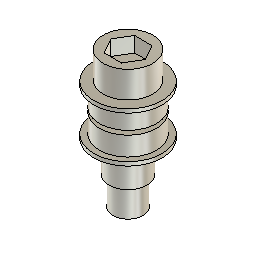
Mark III Core XY assembly v25 (Autodesk Fusion 360 archive; units mm, degrees)
design "8mm pulley low"
Autodesk Fusion 360 part; units mm, degrees
(part 1 of 2)
sketch "Sketch1" plane through (0, 0, 0) normal (0, 0, 1) x (1, 0, 0)
sketch "Sketch2" plane through (0, 0, 0) normal (0, 0, 1) x (1, 0, 0)
  circle A0 centre (0, 0) radius 4
  dimension "d4" = 8
  constraint coincident A0.centre origin
  measures "d4" diameter of A0
extrude "Extrude2" add sketch "Sketch2" along normal blind 27 contours A0 picked at (1.42018, -0.528552) makes body 1
sketch "Sketch3" plane through (0, 0, 27) normal (0, 0, 1) x (-1, 0, 0)
  circle A0 centre (0, 0) radius 4
  circle A1 centre (0, 0) radius 6.5
  dimension "d7" = 13
  constraint concentric A0 A1
  measures "d7" diameter of A1
extrude "Extrude3" add sketch "Sketch3" along normal blind 10 contours A0 | A1 picked at (-0.705317, 0.780795) picked at (5.627575, -0.521648) bodies 1
sketch "Sketch4" plane through (0, 0, 37) normal (0, 0, 1) x (-1, 0, 0)
  circle A0 centre (0, 0) radius 6.5
  line L0 (-4.618187, 0.0754) -> (-2.374392, -3.961767)
  line L1 (-2.374392, -3.961767) -> (2.243795, -4.037167)
  line L2 (2.243795, -4.037167) -> (4.618187, -0.0754)
  line L3 (4.618187, -0.0754) -> (2.374392, 3.961767)
  line L4 (2.374392, 3.961767) -> (-2.243795, 4.037167)
  line L5 (-2.243795, 4.037167) -> (-4.618187, 0.0754)
  dimension "d10" = 4
  constraint coincident A0.centre origin
  measures "d10" distance of A0.centre L5
extrude "Extrude4" cut sketch "Sketch4" against normal blind 7 contours L0 L1 L2 L3 L4 L5 picked at (-1.539396, 0.025133) bodies 1
thread "Thread1" [suppressed]
sketch "Sketch5" plane through (0, 0, 37) normal (0, 0, 1) x (-1, 0, 0)
  circle A0 centre (-1.50985, 25.955849) radius 4
  circle A1 centre (-1.50985, 25.955849) radius 8
  circle A2 centre (-1.50985, 25.955849) radius 9
  dimension "d13" = 8
  dimension "d14" = 16
  dimension "d15" = 18
  constraint concentric A0 A1
  constraint concentric A1 A2
  measures "d13" diameter of A0
  measures "d14" diameter of A1
  measures "d15" diameter of A2
sketch "Sketch6" plane through (0, 0, 42) normal (0, 0, 1) x (-1, 0, 0)
  circle A0 centre (-1.50985, 25.955849) radius 4
  circle A1 centre (-1.50985, 25.955849) radius 8
  circle A2 centre (-1.50985, 25.955849) radius 5
  circle A3 centre (-1.50985, 25.955849) radius 7.5
  dimension "d20" = 10
  dimension "d21" = 15
  constraint concentric A0 A2
  constraint concentric A2 A3
  measures "d20" diameter of A2
  measures "d21" diameter of A3
extrude "Extrude7" add sketch "Sketch6" against normal blind 5 separate body contours A3 picked at (5.110278, 25.33484) makes body 2
extrude "Extrude8" add sketch "Sketch5" against normal blind 1 separate body contours A2 picked at (7.093525, 25.111277) makes body 3
sketch "Sketch7" plane through (0, 0, 42) normal (0, 0, 1) x (1, 0, 0)
extrude "Extrude9" add sketch "Sketch5" against normal blind 1 contours A1 picked at (5.11214, 25.35968) bodies 2 3
move_face "OffsetFaces1" offset 5 1 faces at (-3.138201, -25.707446, 37) on bodies 2
copy_body "CopyPasteBodies1" bodies 2 makes body 4
move_body "Move1" bodies 4 to x (-1, 0, 0) y (0, 1, 0) z (0, 0, -1) at (3.0197, 0, 84.5)
move_body "Move2" bodies 1 to x (1, 0, 0) y (0, 1, 0) z (0, 0, 1) at (44, -25, 0)
move_body "Align1" bodies 1 to x (1, 0, 0) y (0, 1, 0) z (0, 0, 1) at (-42.49015, -0.955849, 45.732394)
move_body "Move3" bodies 2 4 to x (1, 0, 0) y (0, 1, 0) z (0, 0, 1) at (0, 0, 24)
move_body "Move4" bodies 2 to x (1, 0, 0) y (0, 1, 0) z (0, 0, 1) at (0, 0, -55)
sketch "Sketch8" plane through (0, 0, 45.732394) normal (0, 0, -1) x (1, 0, 0)
  circle A0 centre (1.50914, 25.951936) radius 4
  circle A1 centre (1.50914, 25.951936) radius 5
  circle A2 centre (1.50985, 25.955849) radius 4
  dimension "d29" = 8
  dimension "d30" = 10
  constraint concentric A0 A1
  measures "d29" diameter of A0
  measures "d30" diameter of A1
extrude "Extrude10" add sketch "Sketch6" along normal blind 1 separate body contours A2 picked at (3.138201, 25.707446) makes body 5
move_body "Move5" bodies 5 to x (1, 0, 0) y (0, 1, 0) z (0, 0, 1) at (0, 0, 23.5)
move_body "Move6" bodies 2 to x (1, 0, 0) y (0, 1, 0) z (0, 0, 1) at (0, 0, 54.4)
sketch "Sketch9" plane through (0, 0, 45.732394) normal (0, 0, -1) x (1, 0, 0)
  circle A0 centre (1.50974, 25.955286) radius 4
  circle A1 centre (1.50974, 25.955286) radius 5
  circle A2 centre (1.50985, 25.955849) radius 4
  dimension "d34" = 8
  dimension "d35" = 10
  constraint concentric A0 A1
  measures "d34" diameter of A0
  measures "d35" diameter of A1
extrude "Extrude11" add sketch "Sketch8" against normal blind 10 separate body contours A1 picked at (-0.514215, 21.757072) makes body 6
move_body "Move7" bodies 6 to x (1, 0, 0) y (0, 1, 0) z (0, 0, 1) at (0, 0, 3.5)
move_face "OffsetFaces3" offset -3 1 faces at (-0.514215, -21.757072, 49.232394) on bodies 6
extrude "Extrude12" cut 1 faces at (1.715297, -21.12893, 82.732394) along direction (0, 0, -1) blind 3 on bodies 1 bodies 1
move_face "OffsetFaces4" offset 2 1 faces at (2.883587, -26.892448, 45.732394) on bodies 1
extrude "Extrude13" add 1 faces at (-0.514215, -21.757072, 52.232394) along direction (0, 0, -1) blind 1.0883 on bodies 6 bodies 6 2 4 5 1
ref_plane "WorkPlane1" through (0, -2, 0) normal (0, 1, 0) x (0, 0, 1)
sketch "Sketch10" plane through (0, -2, 0) normal (0, 1, 0) x (1, 0, 0)
  line L0 (6.509162, -59.23223) -> (6.509162, -51.144083)
  constraint vertical L0
sketch "Sketch11" plane through (0, 0, 0) normal (0, 1, 0) x (1, 0, 0)
combine "Combine1" [suppressed]
named bodies: "pulley low"

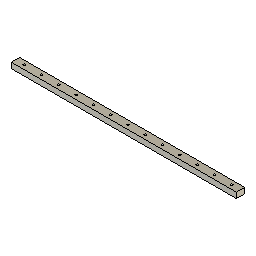
design "rail"
Autodesk Fusion 360 part; units mm, degrees
sketch "Sketch1" plane through (0, 0, 0) normal (0, 0, 1) x (1, 0, 0)
  line L0 (0, 0) -> (325, 0)
  line L1 (325, 0) -> (325, -12)
  line L2 (325, -12) -> (0, -12)
  line L3 (0, -12) -> (0, 0)
  circle A0 centre (12.5, -6) radius 1.5
  circle A1 centre (37.5, -6) radius 1.5
  circle A2 centre (62.5, -6) radius 1.5
  circle A3 centre (87.5, -6) radius 1.5
  circle A4 centre (137.5, -6) radius 1.5
  circle A5 centre (112.5, -6) radius 1.5
  circle A6 centre (262.5, -6) radius 1.5
  circle A7 centre (162.5, -6) radius 1.5
  circle A8 centre (212.5, -6) radius 1.5
  circle A9 centre (237.5, -6) radius 1.5
  circle A10 centre (287.5, -6) radius 1.5
  circle A11 centre (187.5, -6) radius 1.5
  circle A12 centre (312.5, -6) radius 1.5
  point P0 (287.5, -6)
  point P1 (262.5, -6)
  point P2 (187.5, -6)
  point P3 (112.5, -6)
  point P4 (37.5, -6)
  point P5 (62.5, -6)
  point P6 (87.5, -6)
  point P7 (162.5, -6)
  point P8 (137.5, -6)
  point P9 (212.5, -6)
  point P10 (237.5, -6)
  point P11 (12.5, -6)
  point P12 (112.5, -6)
  point P13 (87.5, -6)
  point P14 (137.5, -6)
  point P15 (287.5, -6)
  point P16 (262.5, -6)
  point P17 (187.5, -6)
  point P18 (237.5, -6)
  point P19 (262.5, -6)
  point P20 (287.5, -6)
  point P21 (237.5, -6)
  point P22 (162.5, -6)
  point P23 (212.5, -6)
  point P24 (312.5, -6)
  point P25 (312.5, -6)
  point P26 (312.5, -6)
  dimension "d1" = 325
  dimension "d2" = 12
  dimension "d6" = 25
  dimension "d12" = 25
  dimension "d13" = 25
  dimension "d14" = 25
  dimension "d15" = 25
  dimension "d16" = 25
  dimension "d17" = 25
  dimension "d18" = 25
  dimension "d19" = 3
  dimension "d20" = 3
  dimension "d21" = 3
  dimension "d22" = 25
  dimension "d23" = 25
  dimension "d24" = 3
  dimension "d25" = 3
  dimension "d26" = 3
  dimension "d27" = 25
  dimension "d28" = 25
  dimension "d29" = 25
  dimension "d30" = 25
  dimension "d31" = 3
  dimension "d32" = 3
  dimension "d33" = 3
  dimension "d34" = 25
  dimension "d35" = 25
  dimension "d36" = 3
  dimension "d37" = 3
  dimension "d38" = 3
  dimension "d39" = 3
  constraint horizontal L0
  constraint vertical L1
  constraint horizontal L2
  constraint vertical L3
  constraint coincident L0.start L3.end
  constraint coincident P11 A0.centre
  constraint coincident P4 A1.centre
  constraint coincident P5 A2.centre
  constraint coincident P13 P6
  constraint coincident P12 P3
  constraint coincident P14 P8
  constraint coincident P22 P7
  constraint coincident P17 P2
  constraint coincident P23 P9
  constraint coincident P21 P18
  constraint coincident P19 P16
  constraint coincident P20 P15
  constraint coincident P26 P25
  measures "d1" distance of L0.start L0.end
  measures "d2" distance of L0.start L2.end
  measures "d6" distance of P20 P19
  measures "d12" distance of P4 P5
  measures "d13" distance of P5 P13
  measures "d14" distance of P12 P14
  measures "d15" distance of P22 P14
  measures "d16" distance of P17 P23
  measures "d17" distance of P23 P21
  measures "d18" distance of P4 P11
  measures "d19" diameter of A0
  measures "d20" diameter of A1
  measures "d21" diameter of A2
  measures "d22" distance of P12 P14
  measures "d23" distance of P12 P13
  measures "d24" diameter of A3
  measures "d25" diameter of A5
  measures "d26" diameter of A4
  measures "d27" distance of P17 P23
  measures "d28" distance of P21 P23
  measures "d29" distance of P20 P19
  measures "d30" distance of P17 P22
  measures "d31" diameter of A7
  measures "d32" diameter of A11
  measures "d33" diameter of A8
  measures "d34" distance of P19 P20
  measures "d35" distance of P21 P19
  measures "d36" diameter of A9
  measures "d37" diameter of A6
  measures "d38" diameter of A10
  measures "d39" diameter of A12
extrude "Extrude1" add sketch "Sketch1" along normal blind 8

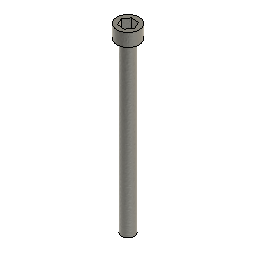
design "long stepper allen bolt"
Autodesk Fusion 360 part; units mm, degrees
sketch "Sketch1" plane through (0, 0, 0) normal (0, 0, 1) x (1, 0, 0)
  circle A0 centre (0, 0) radius 2.5
  dimension "d1" = 5
  constraint coincident A0.centre origin
  measures "d1" diameter of A0
extrude "Extrude1" add sketch "Sketch1" along normal blind 65
sketch "Sketch2" plane through (0, 0, 65) normal (0, 0, 1) x (-1, 0, 0)
  circle A0 centre (0, 0) radius 2.5
  circle A1 centre (0, 0) radius 4.3
  dimension "d4" = 8.6
  constraint coincident A0.centre A1.centre
  measures "d4" diameter of A1
extrude "Extrude2" add sketch "Sketch2" along normal blind 5 contours A0 | A1
sketch "Sketch3" plane through (0, 0, 70) normal (0, 0, 1) x (-1, 0, 0)
  circle A0 centre (0, 0) radius 4.3
  line L0 (-2.8697, 0.3419) -> (-1.7309, -2.3143)
  line L1 (-1.7309, -2.3143) -> (1.1388, -2.6561)
  line L2 (1.1388, -2.6561) -> (2.8697, -0.3419)
  line L3 (2.8697, -0.3419) -> (1.7309, 2.3143)
  line L4 (1.7309, 2.3143) -> (-1.1388, 2.6561)
  line L5 (-1.1388, 2.6561) -> (-2.8697, 0.3419)
  dimension "d7" = 2.5028
  constraint coincident A0.centre origin
  measures "d7" distance of A0.centre L5
extrude "Extrude3" cut sketch "Sketch3" against normal blind 4 contours L0 L1 L2 L3 L4 L5

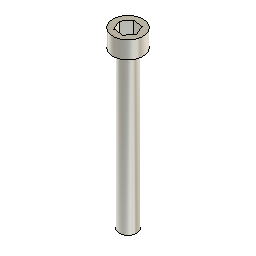
design "45mm short  stepper allen bolt"
Autodesk Fusion 360 part; units mm, degrees
sketch "Sketch1" plane through (0, 0, 0) normal (0, 0, 1) x (1, 0, 0)
  circle A0 centre (0, 0) radius 2.5
  dimension "d1" = 5
  constraint coincident A0.centre origin
  measures "d1" diameter of A0
sketch "Sketch2" plane through (0, 0, 65) normal (0, 0, 1) x (-1, 0, 0)
  circle A0 centre (0, 0) radius 2.5
  circle A1 centre (0, 0) radius 4.3
  dimension "d4" = 8.6
  constraint coincident A0.centre A1.centre
  measures "d4" diameter of A1
extrude "Extrude4" add sketch "Sketch1" along normal blind 45 makes body 1
extrude "Extrude2" add sketch "Sketch2" along normal blind 5 contours A0 | A1 makes body 2
sketch "Sketch3" plane through (0, 0, 70) normal (0, 0, 1) x (-1, 0, 0)
  circle A0 centre (0, 0) radius 4.3
  line L0 (-2.8697, 0.3419) -> (-1.7309, -2.3143)
  line L1 (-1.7309, -2.3143) -> (1.1388, -2.6561)
  line L2 (1.1388, -2.6561) -> (2.8697, -0.3419)
  line L3 (2.8697, -0.3419) -> (1.7309, 2.3143)
  line L4 (1.7309, 2.3143) -> (-1.1388, 2.6561)
  line L5 (-1.1388, 2.6561) -> (-2.8697, 0.3419)
  dimension "d7" = 2.5028
  constraint coincident A0.centre origin
  measures "d7" distance of A0.centre L5
extrude "Extrude3" cut sketch "Sketch3" against normal blind 4 contours L0 L1 L2 L3 L4 L5 bodies 2
move_body "Align1" bodies 2 to x (1, 0, 0) y (0, 1, 0) z (0, 0, 1) at (0, 0, -20)

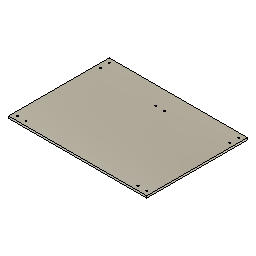
design "bottom plate"
Autodesk Fusion 360 part; units mm, degrees
sketch "Sketch1" plane through (0, 0, 0) normal (0, 0, 1) x (1, 0, 0)
  line L0 (14.0053, -24.8588) -> (645.8303, -24.8588)
  line L1 (645.8303, -24.8588) -> (645.8303, -485.2338)
  line L2 (645.8303, -485.2338) -> (14.0053, -485.2338)
  line L3 (14.0053, -485.2338) -> (14.0053, -24.8588)
  dimension "d1" = 631.825
  dimension "d2" = 460.375
  constraint horizontal L0
  constraint vertical L1
  constraint horizontal L2
  constraint vertical L3
  measures "d1" distance of L0.start L0.end
  measures "d2" distance of L0.start L2.end
extrude "Extrude1" add sketch "Sketch1" along normal blind 9.525
sketch "Sketch2" plane through (0, 0, 19.05) normal (0, 0, 1) x (-1, 0, 0)
  circle A0 centre (-559.9411, 33.0388) radius 2
  circle A1 centre (-607.0811, 33.0388) radius 2
  circle A2 centre (-610.8303, 63.0463) radius 3.5
  circle A3 centre (-48.9178, 458.0463) radius 3.5
  circle A4 centre (-610.9178, 458.0463) radius 3.5
  circle A5 centre (-349.9178, 108.3588) radius 3.5
  circle A6 centre (-309.9178, 108.3588) radius 3.5
  circle A7 centre (-625.8303, 84.8588) radius 3.5
  circle A8 centre (-625.8303, 44.8588) radius 3.5
  circle A9 centre (-34.0053, 84.8588) radius 3.5
  circle A10 centre (-34.0053, 44.8588) radius 3.5
  circle A11 centre (-594.8678, 98.3622) radius 3.5
  circle A12 centre (-48.9178, 63.0463) radius 3.5
  circle A13 centre (-76.3246, 82.1788) radius 3.5
  circle A14 centre (-583.5111, 82.1788) radius 3.5
  circle A15 centre (-64.9678, 98.3204) radius 3.5
  circle A16 centre (-625.8303, 465.2338) radius 3.5
  circle A17 centre (-585.8303, 465.2338) radius 3.5
  circle A18 centre (-74.0053, 465.2338) radius 3.5
  circle A19 centre (-34.0053, 465.2338) radius 3.5
  circle A20 centre (-559.9411, 80.1788) radius 2
  circle A21 centre (-607.0811, 80.1788) radius 2
  circle A22 centre (-583.5111, 56.6088) radius 3.5
  circle A23 centre (-99.8946, 80.1788) radius 2
  circle A24 centre (-99.8946, 33.0388) radius 2
  circle A25 centre (-76.3246, 56.6088) radius 3.5
  circle A26 centre (-52.7546, 33.0388) radius 2
  line L0 (-14.0053, 24.8588) -> (-14.0053, 485.2338)
  line L1 (-14.0053, 485.2338) -> (-94.0053, 485.2338)
  line L2 (-94.0053, 485.2338) -> (-94.0053, 445.2338)
  line L3 (-94.0053, 445.2338) -> (-92.5053, 445.2338)
  arc A27 (-77.5053, 430.2338) -> (-92.5053, 445.2338) centre (-92.5053, 430.2338) ccw
  line L4 (-77.5053, 430.2338) -> (-77.5053, 108.3588)
  arc A28 (-97.5053, 88.3588) -> (-77.5053, 108.3588) centre (-97.5053, 108.3588) ccw
  line L5 (-97.5053, 88.3588) -> (-269.9178, 88.3588)
  arc A29 (-289.9178, 108.3588) -> (-269.9178, 88.3588) centre (-269.9178, 108.3588) ccw
  line L6 (-289.9178, 108.3588) -> (-289.9178, 128.3588)
  line L7 (-289.9178, 128.3588) -> (-369.9178, 128.3588)
  line L8 (-369.9178, 128.3588) -> (-369.9178, 108.3588)
  arc A30 (-389.9178, 88.3588) -> (-369.9178, 108.3588) centre (-389.9178, 108.3588) ccw
  line L9 (-389.9178, 88.3588) -> (-562.3303, 88.3588)
  arc A31 (-582.3303, 108.3588) -> (-562.3303, 88.3588) centre (-562.3303, 108.3588) ccw
  line L10 (-582.3303, 108.3588) -> (-582.3303, 430.2338)
  arc A32 (-567.3303, 445.2338) -> (-582.3303, 430.2338) centre (-567.3303, 430.2338) ccw
  line L11 (-567.3303, 445.2338) -> (-565.8303, 445.2338)
  line L12 (-565.8303, 445.2338) -> (-565.8303, 485.2338)
  line L13 (-565.8303, 485.2338) -> (-645.8303, 485.2338)
  line L14 (-645.8303, 485.2338) -> (-645.8303, 24.8588)
  line L15 (-645.8303, 24.8588) -> (-14.0053, 24.8588)
  point P0 (-34.0053, 44.8588)
  point P1 (-34.0053, 84.8588)
  point P2 (-349.9178, 108.3588)
  point P3 (-309.9178, 108.3588)
  point P4 (-625.8303, 84.8588)
  point P5 (-625.8303, 44.8588)
  point P6 (-625.8303, 465.2338)
  point P7 (-585.8303, 465.2338)
  point P8 (-34.0053, 465.2338)
  point P9 (-74.0053, 465.2338)
  constraint coincident P0 A10.centre
  constraint coincident P1 A9.centre
  constraint coincident P2 A5.centre
  constraint coincident P3 A6.centre
  constraint coincident P4 A7.centre
  constraint coincident P5 A8.centre
  constraint coincident P6 A16.centre
  constraint coincident P7 A17.centre
  constraint coincident P8 A19.centre
  constraint coincident P9 A18.centre
hole "Hole1" at (34.0053, -465.2338, 19.05) direction (0, 0, -1) diameter 7 depth 60 tip angle 118
hole "Hole2" at (74.0053, -465.2338, 19.05) at (34.0053, -44.8588, 19.05) at (34.0053, -84.8588, 19.05) at (625.8303, -44.8588, 19.05) at (625.8303, -84.8588, 19.05) direction (0, 0, -1) diameter 7 depth 60 tip angle 118
hole "Hole3" at (625.8303, -465.2338, 19.05) at (585.8303, -465.2338, 19.05) direction (0, 0, -1) diameter 7 depth 60 tip angle 118
hole "Hole4" at (309.9178, -108.3588, 19.05) at (349.9178, -108.3588, 19.05) direction (0, 0, -1) diameter 7 depth 60 tip angle 118

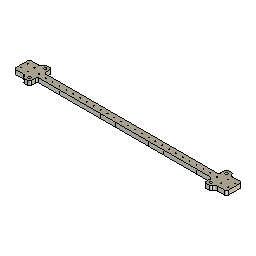
design "Mark III core xy  bridge"
Autodesk Fusion 360 part; units mm, degrees
sketch "Sketch2" plane through (0, 0, 0) normal (0, 0, 1) x (1, 0, 0)
sketch "Sketch5" plane through (0, 0, 9.525) normal (0, 0, 1) x (-1, 0, 0)
sketch "Sketch30" plane through (0, 0, 9.525) normal (0, 0, 1) x (-1, 0, 0)
  line L0 (-255, 10) -> (255, 10)
  line L1 (255, -10) -> (-255, -10)
  line L2 (275, 22.5) -> (310, 22.5)
  line L3 (310, 22.5) -> (310, -22.5)
  line L4 (310, -22.5) -> (275, -22.5)
  line L5 (-310, 22.5) -> (-275, 22.5)
  line L6 (-275, -22.5) -> (-310, -22.5)
  line L7 (-310, -22.5) -> (-310, 22.5)
  line L8 (-275, 22.5) -> (-275, 27.5)
  line L9 (-270, 32.5) -> (-260, 32.5)
  line L10 (-255, 27.5) -> (-255, 10)
  line L11 (-275, -22.5) -> (-275, -27.5)
  line L12 (-270, -32.5) -> (-260, -32.5)
  line L13 (-255, -27.5) -> (-255, -10)
  line L14 (275, -22.5) -> (275, -27.5)
  line L15 (270, -32.5) -> (260, -32.5)
  line L16 (255, -27.5) -> (255, -10)
  line L17 (275, 22.5) -> (275, 27.5)
  line L18 (270, 32.5) -> (260, 32.5)
  line L19 (255, 27.5) -> (255, 10)
  arc A0 (-260, -32.5) -> (-255, -27.5) centre (-260, -27.5) ccw
  arc A1 (-255, 27.5) -> (-260, 32.5) centre (-260, 27.5) ccw
  arc A2 (255, -27.5) -> (260, -32.5) centre (260, -27.5) ccw
  arc A3 (260, 32.5) -> (255, 27.5) centre (260, 27.5) ccw
  arc A4 (275, 27.5) -> (270, 32.5) centre (270, 27.5) ccw
  arc A5 (270, -32.5) -> (275, -27.5) centre (270, -27.5) ccw
  arc A6 (-275, -27.5) -> (-270, -32.5) centre (-270, -27.5) ccw
  arc A7 (-270, 32.5) -> (-275, 27.5) centre (-270, 27.5) ccw
  point P0 (292.5, 0)
  point P1 (-292.5, 0)
  point P2 (-20, 0)
  point P3 (-40, 0)
  point P4 (-100, 0)
  point P5 (-60, 0)
  point P6 (-80, 0)
  point P7 (-60, 0)
  point P8 (-160, 0)
  point P9 (-120, 0)
  point P10 (-220, 0)
  point P11 (-180, 0)
  point P12 (-140, 0)
  point P13 (-200, 0)
  point P14 (-120, 0)
  point P15 (-180, 0)
  point P16 (-240, 0)
  point P17 (-220, 0)
  point P18 (-220, 0)
  point P19 (220, 0)
  point P20 (260, 0)
  point P21 (120, 0)
  point P22 (40, 0)
  point P23 (160, 0)
  point P24 (200, 0)
  point P25 (240, 0)
  point P26 (180, 0)
  point P27 (260, 0)
  point P28 (20, 0)
  point P29 (40, 0)
  point P30 (200, 0)
  point P31 (60, 0)
  point P32 (140, 0)
  point P33 (80, 0)
  point P34 (40, 0)
  point P35 (100, 0)
  point P36 (140, 0)
  point P37 (80, 0)
  point P38 (240, 0)
  point P39 (220, 0)
  point P40 (180, 0)
  point P41 (160, 0)
  point P42 (120, 0)
  point P43 (100, 0)
  point P44 (60, 0)
  point P45 (20, 0)
  point P46 (-80, 0)
  point P47 (-100, 0)
  point P48 (-140, 0)
  point P49 (-160, 0)
  point P50 (-200, 0)
  point P51 (-240, 0)
  point P52 (-260, 0)
  point P53 (-260, 0)
  point P54 (292.5, 0)
  point P55 (282.5, -10)
  point P56 (302.5, -10)
  point P57 (302.5, 10)
  point P58 (282.5, 10)
  point P59 (-302.5, -10)
  point P60 (-282.5, -10)
  point P61 (-282.5, 10)
  point P62 (-302.5, 10)
  point P63 (-275, 32.5)
  point P64 (-255, 32.5)
  point P65 (-275, -32.5)
  point P66 (-255, -32.5)
  point P67 (275, -32.5)
  point P68 (255, -32.5)
  point P69 (275, 32.5)
  point P70 (255, 32.5)
  dimension "d349" = 35
  dimension "d350" = 45
  dimension "d351" = 35
  dimension "d352" = 45
  dimension "d353" = 20
  dimension "d354" = 20
  dimension "d355" = 20
  dimension "d356" = 20
  dimension "d357" = 20
  dimension "d358" = 20
  dimension "d359" = 20
  dimension "d360" = 20
  dimension "d361" = 20
  dimension "d363" = 20
  dimension "d364" = 20
  dimension "d365" = 20
  dimension "d366" = 20
  dimension "d367" = 20
  dimension "d368" = 20
  dimension "d369" = 20
  dimension "d370" = 20
  dimension "d371" = 20
  dimension "d372" = 20
  dimension "d373" = 20
  dimension "d374" = 20
  dimension "d375" = 20
  dimension "d376" = 10
  dimension "d377" = 20
  dimension "d378" = 10
  dimension "d379" = 20
  dimension "d380" = 10
  dimension "d381" = 20
  dimension "d382" = 10
  dimension "d383" = 20
  dimension "d384" = 5
  dimension "d385" = 5
  constraint parallel L0 L1
  constraint horizontal L0
  constraint perpendicular L2 L3
  constraint parallel L2 L4
  constraint horizontal L2
  constraint parallel L5 L6
  constraint horizontal L5
  constraint coincident P7 P5
  constraint coincident P14 P9
  constraint coincident P15 P11
  constraint coincident P18 P17
  constraint coincident P27 P20
  constraint coincident P30 P24
  constraint coincident P36 P32
  constraint coincident P37 P33
  constraint coincident P34 P29
  constraint coincident P38 P25
  constraint coincident P39 P19
  constraint coincident P40 P26
  constraint coincident P41 P23
  constraint coincident P42 P21
  constraint coincident P43 P35
  constraint coincident P44 P31
  constraint coincident P45 P28
  constraint coincident P46 P6
  constraint coincident P47 P4
  constraint coincident P48 P12
  constraint coincident P49 P8
  constraint coincident P50 P13
  constraint coincident P51 P16
  constraint coincident P53 P52
  constraint coincident P54 P0
  constraint perpendicular L5 L8
  constraint perpendicular L8 L9
  constraint perpendicular L0 L10
  constraint perpendicular L6 L11
  constraint perpendicular L11 L12
  constraint perpendicular L1 L13
  constraint perpendicular L4 L14
  constraint perpendicular L14 L15
  constraint perpendicular L1 L16
  constraint perpendicular L1 L17
  constraint perpendicular L17 L18
  constraint perpendicular L0 L19
  constraint coincident P66 L12
  constraint coincident P66 L13
  constraint tangent L12 A0
  constraint tangent L13 A0
  constraint coincident P64 L9
  constraint coincident P64 L10
  constraint tangent L9 A1
  constraint tangent L10 A1
  constraint coincident P68 L15
  constraint coincident P68 L16
  constraint tangent L15 A2
  constraint tangent L16 A2
  constraint equal A1 A2
  constraint coincident P70 L18
  constraint coincident P70 L19
  constraint tangent L18 A3
  constraint tangent L19 A3
  constraint equal A1 A3
  constraint coincident P69 L17
  constraint coincident P69 L18
  constraint tangent L17 A4
  constraint tangent L18 A4
  constraint equal A1 A4
  constraint coincident P67 L14
  constraint coincident P67 L15
  constraint tangent L14 A5
  constraint tangent L15 A5
  constraint equal A1 A5
  constraint coincident P65 L11
  constraint coincident P65 L12
  constraint tangent L11 A6
  constraint tangent L12 A6
  constraint equal A1 A6
  constraint coincident P63 L8
  constraint coincident P63 L9
  constraint tangent L8 A7
  constraint tangent L9 A7
  constraint equal A1 A7
  measures "d349" distance of L3.end L4.end
  measures "d350" distance of L2.end L3.end
  measures "d351" distance of L6.start L6.end
  measures "d352" distance of L5.end L6.start
  measures "d353" distance of origin P2
  measures "d354" distance of P2 P3
  measures "d355" distance of P7 P46
  measures "d356" distance of P47 P46
  measures "d357" distance of P14 P48
  measures "d358" distance of P49 P48
  measures "d359" distance of P15 P50
  measures "d360" distance of P18 P50
  measures "d361" distance of P51 P18
  measures "d363" distance of P27 P38
  measures "d364" distance of P39 P38
  measures "d365" distance of P30 P40
  measures "d366" distance of P41 P40
  measures "d367" distance of P42 P36
  measures "d368" distance of P42 P43
  measures "d369" distance of P44 P37
  measures "d370" distance of P31 P34
  measures "d371" distance of P34 P45
  measures "d372" distance of P55 P56
  measures "d373" distance of P56 P57
  measures "d374" distance of P59 P60
  measures "d375" distance of P60 P61
  measures "d376" distance of L5.end P63
  measures "d377" distance of P63 P64
  measures "d378" distance of L6.start P65
  measures "d379" distance of P65 P66
  measures "d380" distance of L4.end P67
  measures "d381" distance of P67 P68
  measures "d382" distance of L2.start P69
  measures "d383" distance of P69 P70
  measures "d384" radius of A0
  measures "d385" radius of A1
extrude "Extrude17" add sketch "Sketch30" along normal blind 12.7 makes body 1
hole "Hole31" at (-265, -23, 0) direction (0, 0, 1) diameter 7 depth 200 tip angle 118 bodies 1
hole "Hole32" at (-264.95, 22.9974, 0) direction (0, 0, 1) diameter 7 depth 200 tip angle 118 bodies 1
hole "Hole33" at (265, -22.9937, 0) at (265, 23, 0) direction (0, 0, 1) diameter 7 depth 200 tip angle 118 bodies 1
hole "Hole34" at (-302.5, -10, 9.525) direction (0, 0, 1) diameter 3 depth 200 tip angle 118 bodies 1
hole "Hole35" at (-302.5, 10, 9.525) at (-282.5, 10, 9.525) at (-282.5, -10, 9.525) at (302.5, -10, 9.525) at (282.5, -10, 9.525) at (282.5, 10, 9.525) at (302.5, 10, 9.525) direction (0, 0, 1) diameter 3 depth 200 tip angle 118 bodies 1
hole "Hole36" at (260, 0, 9.525) direction (0, 0, 1) diameter 2.5 depth 200 tip angle 118 bodies 1
hole "Hole37" at (240, 0, 9.525) at (220, 0, 9.525) at (200, 0, 9.525) at (180, 0, 9.525) at (160, 0, 9.525) at (140, 0, 9.525) at (120, 0, 9.525) at (100, 0, 9.525) at (80, 0, 9.525) at (60, 0, 9.525) at (40, 0, 9.525) at (20, 0, 9.525) at (-20, 0, 9.525) at (-40, 0, 9.525) at (-60, 0, 9.525) at (-80, 0, 9.525) at (-100, 0, 9.525) at (-260, 0, 9.525) at (-240, 0, 9.525) at (-220, 0, 9.525) at (-200, 0, 9.525) at (-180, 0, 9.525) at (-160, 0, 9.525) at (-140, 0, 9.525) at (-120, 0, 9.525) direction (0, 0, 1) diameter 2.5 depth 200 tip angle 118 bodies 1
hole "Hole38" at (0, 0, 9.525) direction (0, 0, 1) diameter 2.5 depth 200 tip angle 118 bodies 1
thread "Thread1" [suppressed]
fillet "Fillet1" radius 5 4 edges at (-310, 22.5, 15.875) (310, 22.5, 15.875) (310, -22.5, 15.875) (-310, -22.5, 15.875) on bodies 1
fillet "Fillet2" radius 5 4 edges at (-255, -10, 15.875) (255, -10, 15.875) (-255, 10, 15.875) (255, 10, 15.875) on bodies 1
move_body "Move32" bodies 1 to x (1, 0, 0) y (0, 1, 0) z (0, 0, 1) at (0, 0, 20)
sketch "Sketch31" plane through (0, 0, 29.525) normal (0, 0, -1) x (1, 0, 0)
  arc A0 (-305, 22.5) -> (-310, 17.5) centre (-305, 17.5) ccw
  line L0 (-310, 17.5) -> (-310, -17.5)
  arc A1 (-310, -17.5) -> (-305, -22.5) centre (-305, -17.5) ccw
  line L1 (-305, -22.5) -> (-275, -22.5)
  line L2 (-275, -22.5) -> (-275, -27.5)
  arc A2 (-275, -27.5) -> (-270, -32.5) centre (-270, -27.5) ccw
  line L3 (-270, -32.5) -> (-260, -32.5)
  arc A3 (-260, -32.5) -> (-255, -27.5) centre (-260, -27.5) ccw
  line L4 (-255, -27.5) -> (-255, -15)
  arc A4 (-250, -10) -> (-255, -15) centre (-250, -15) ccw
  line L5 (-250, -10) -> (250, -10)
  arc A5 (255, -15) -> (250, -10) centre (250, -15) ccw
  line L6 (255, -15) -> (255, -27.5)
  arc A6 (255, -27.5) -> (260, -32.5) centre (260, -27.5) ccw
  line L7 (260, -32.5) -> (270, -32.5)
  arc A7 (270, -32.5) -> (275, -27.5) centre (270, -27.5) ccw
  line L8 (275, -27.5) -> (275, -22.5)
  line L9 (275, -22.5) -> (305, -22.5)
  arc A8 (305, -22.5) -> (310, -17.5) centre (305, -17.5) ccw
  line L10 (310, -17.5) -> (310, 17.5)
  arc A9 (310, 17.5) -> (305, 22.5) centre (305, 17.5) ccw
  line L11 (305, 22.5) -> (275, 22.5)
  line L12 (275, 22.5) -> (275, 27.5)
  arc A10 (275, 27.5) -> (270, 32.5) centre (270, 27.5) ccw
  line L13 (270, 32.5) -> (260, 32.5)
  arc A11 (260, 32.5) -> (255, 27.5) centre (260, 27.5) ccw
  line L14 (255, 27.5) -> (255, 15)
  arc A12 (250, 10) -> (255, 15) centre (250, 15) ccw
  line L15 (250, 10) -> (-250, 10)
  arc A13 (-255, 15) -> (-250, 10) centre (-250, 15) ccw
  line L16 (-255, 15) -> (-255, 27.5)
  arc A14 (-255, 27.5) -> (-260, 32.5) centre (-260, 27.5) ccw
  line L17 (-260, 32.5) -> (-270, 32.5)
  arc A15 (-270, 32.5) -> (-275, 27.5) centre (-270, 27.5) ccw
  line L18 (-275, 27.5) -> (-275, 22.5)
  line L19 (-275, 22.5) -> (-305, 22.5)
  circle A16 centre (0, 0) radius 1.25
  circle A17 centre (-140, 0) radius 1.25
  circle A18 centre (-180, 0) radius 1.25
  circle A19 centre (-220, 0) radius 1.25
  circle A20 centre (-260, 0) radius 1.25
  circle A21 centre (-80, 0) radius 1.25
  circle A22 centre (-40, 0) radius 1.25
  circle A23 centre (20, 0) radius 1.25
  circle A24 centre (60, 0) radius 1.25
  circle A25 centre (100, 0) radius 1.25
  circle A26 centre (140, 0) radius 1.25
  circle A27 centre (180, 0) radius 1.25
  circle A28 centre (220, 0) radius 1.25
  circle A29 centre (240, 0) radius 1.25
  circle A30 centre (200, 0) radius 1.25
  circle A31 centre (160, 0) radius 1.25
  circle A32 centre (120, 0) radius 1.25
  circle A33 centre (80, 0) radius 1.25
  circle A34 centre (40, 0) radius 1.25
  circle A35 centre (-20, 0) radius 1.25
  circle A36 centre (-60, 0) radius 1.25
  circle A37 centre (-100, 0) radius 1.25
  circle A38 centre (-240, 0) radius 1.25
  circle A39 centre (-200, 0) radius 1.25
  circle A40 centre (-160, 0) radius 1.25
  circle A41 centre (-120, 0) radius 1.25
  circle A42 centre (260, 0) radius 1.25
  circle A43 centre (282.5, -10) radius 1.5
  circle A44 centre (302.5, 10) radius 1.5
  circle A45 centre (-282.5, -10) radius 1.5
  circle A46 centre (-302.5, -10) radius 1.5
  circle A47 centre (-282.5, 10) radius 1.5
  circle A48 centre (282.5, 10) radius 1.5
  circle A49 centre (302.5, -10) radius 1.5
  circle A50 centre (-302.5, 10) radius 1.5
  line L20 (249.1231, 8) -> (252.8769, 8)
  line L21 (254.7575, -4.9701) -> (256.7575, 3.0299)
  line L22 (245.2425, 4.9701) -> (243.2425, -3.0299)
  line L23 (247.1231, -8) -> (250.8769, -8)
  arc A51 (249.1231, 8) -> (245.2425, 4.9701) centre (249.1231, 4) ccw
  arc A52 (256.7575, 3.0299) -> (252.8769, 8) centre (252.8769, 4) ccw
  arc A53 (243.2425, -3.0299) -> (247.1231, -8) centre (247.1231, -4) ccw
  arc A54 (250.8769, -8) -> (254.7575, -4.9701) centre (250.8769, -4) ccw
  circle A55 centre (265, 22.9937) radius 3.5
  circle A56 centre (265, -23) radius 3.5
  circle A57 centre (-264.95, -22.9974) radius 3.5
  circle A58 centre (-265, 23) radius 3.5
  point P0 (250, 0)
  dimension "d415" = 4
  dimension "d416" = 4
  dimension "d417" = 4
  dimension "d418" = 4
  constraint horizontal L23
  constraint tangent L22 A51
  constraint tangent L20 A51
  constraint tangent L20 A52
  constraint tangent L21 A52
  constraint tangent L22 A53
  constraint tangent L23 A53
  constraint tangent L21 A54
  constraint tangent L23 A54
  measures "d415" radius of A51
  measures "d416" radius of A52
  measures "d417" radius of A53
  measures "d418" radius of A54
extrude "Extrude18" add sketch "Sketch31" against normal blind 10 separate body contours L20 L21 L22 L23 A51 A52 A53 A54 makes body 2
extrude "Extrude19" add sketch "Sketch31" along normal blind 1 contours L20 L21 L22 L23 A51 A52 A53 A54 bodies 2
copy_body "CopyPasteBodies23" bodies 2 makes body 3
move_body "Move33" bodies 3 to x (1, 0, 0) y (0, 1, 0) z (0, 0, 1) at (-20, 0, 0)
copy_body "CopyPasteBodies24" bodies 3 2 makes body 4 makes body 5
move_body "Move34" bodies 4 5 to x (1, 0, 0) y (0, 1, 0) z (0, 0, 1) at (-40, 0, 0)
copy_body "CopyPasteBodies25" bodies 5 4 3 2 makes body 6 makes body 7 makes body 8 makes body 9
move_body "Move35" bodies 6 7 8 9 to x (1, 0, 0) y (0, 1, 0) z (0, 0, 1) at (-80, 0, 0)
copy_body "CopyPasteBodies26" bodies 9 8 7 6 5 4 3 2 makes body 10 makes body 11 makes body 12 makes body 13 makes body 14 makes body 15 makes body 16 makes body 17
move_body "Move36" bodies 10 11 12 13 14 15 16 17 to x (1, 0, 0) y (0, 1, 0) z (0, 0, 1) at (-160, 0, 0)
copy_body "CopyPasteBodies27" bodies 17 16 15 14 13 12 11 10 makes body 18 makes body 19 makes body 20 makes body 21 makes body 22 makes body 23 makes body 24 makes body 25
move_body "Move37" bodies 18 19 20 21 22 23 24 25 to x (1, 0, 0) y (0, 1, 0) z (0, 0, 1) at (-160, 0, 0)
copy_body "CopyPasteBodies28" bodies 23 makes body 26
move_body "Move38" bodies 26 to x (1, 0, 0) y (0, 1, 0) z (0, 0, 1) at (-20, 0, 0)
copy_body "CopyPasteBodies29" bodies 24 makes body 27
move_body "Move39" bodies 27 to x (1, 0, 0) y (0, 1, 0) z (0, 0, 1) at (-80, 0, 0)
combine "Combine3" operation cut target body 25 tool bodies 2 3 4 5 6 7 8 9 10 11 12 13 14 15 16 17 18 19 20 21 22 23 24 26 27 keep tools
move_face "OffsetFaces7" offset 2 26 faces at (-112.2525, 1.01, 28.525) (-92.2525, 1.01, 28.525) (-192.2525, 1.01, 28.525) (-212.2525, 1.01, 28.525) (-72.2525, 1.01, 28.525) (-132.2525, 1.01, 28.525) (127.7475, 1.01, 28.525) (107.7475, 1.01, 28.525) (187.7475, 1.01, 28.525) (207.7475, 1.01, 28.525) (227.7475, 1.01, 28.525) (247.7475, 1.01, 28.525) (-152.2525, 1.01, 28.525) (-172.2525, 1.01, 28.525) (-252.2525, 1.01, 28.525) (-232.2525, 1.01, 28.525) (7.7475, 1.01, 28.525) (-12.2525, 1.01, 28.525) (-52.2525, 1.01, 28.525) (-32.2525, 1.01, 28.525) (147.7475, 1.01, 28.525) (167.7475, 1.01, 28.525) (27.7475, 1.01, 28.525) (67.7475, 1.01, 28.525) (87.7475, 1.01, 28.525) (47.7475, 1.01, 28.525) on bodies 2 3 4 5 6 7 8 9 10 11 12 13 14 15 16 17 18 19 20 21 22 23 24 25 26 27
combine "Combine9" operation cut target body 1 tool bodies 27 26 23 22 24 25 20 21 19 18 12 13 11 10 15 14 16 17 7 6 8 9 4 5 3 2
fillet "Fillet6" radius 8 1 edges at (275, 22.5, 35.875) on bodies 1
fillet "Fillet7" radius 8 1 edges at (275, -22.5, 35.875) on bodies 1
fillet "Fillet8" radius 8 1 edges at (-275, -22.5, 35.875) on bodies 1
fillet "Fillet9" radius 8 1 edges at (-275, 22.5, 35.875) on bodies 1
named bodies: "bridge", "tool", "tool (1)", "tool (2)", "tool (1) (1)", "tool (2) (1)", "tool (1) (2)", "tool (3)", "tool (1) (1) (1)", "tool (3) (1)", "tool (1) (2) (1)", "tool (2) (1) (1)", "tool (2) (2)", "tool (1) (1) (2)", "tool (1) (3)", "tool (4)", "tool (1) (1) (1) (1)", "tool (4) (1)", "tool (1) (3) (1)", "tool (1) (1) (2) (1)", "tool (2) (2) (1)", "tool (2) (1) (1) (1)", "tool (1) (2) (1) (1)", "tool (3) (1) (1)", "tool (1) (1) (1) (1) (1)", "tool (1) (1) (1) (1) (1) (1)", "tool (1) (2) (1) (1) (1)"

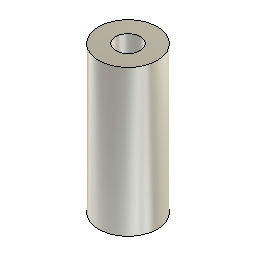
design "short stepper tube"
Autodesk Fusion 360 part; units mm, degrees
sketch "Sketch1" plane through (0, 0, 0) normal (0, 0, 1) x (1, 0, 0)
  circle A0 centre (0, 0) radius 6
  circle A1 centre (0, 0) radius 2.5
  dimension "d1" = 12
  dimension "d2" = 5
  constraint coincident A0.centre A1.centre
  measures "d1" diameter of A0
  measures "d2" diameter of A1
extrude "Extrude2" add sketch "Sketch1" along normal blind 30
ref_plane "WorkPlane1" through (0, 0, 0) normal (0, 1, 0) x (0, 0, 1)
sketch "Sketch2" plane through (0, 0, 0) normal (0, 1, 0) x (1, 0, 0)
  line L0 (-6, -30) -> (-6, 0)
  dimension "d8" = 30
  constraint vertical L0
  measures "d8" distance of L0.start L0.end
extrude "Extrude1" [suppressed]

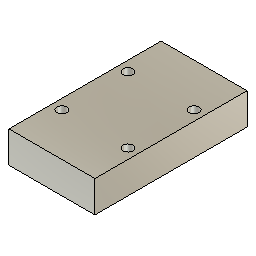
design "bridge block"
Autodesk Fusion 360 part; units mm, degrees
sketch "Sketch1" plane through (0, 0, 0) normal (0, 0, 1) x (1, 0, 0)
  line L0 (13, -23) -> (-13, -23)
  line L1 (-13, -23) -> (-13, 23)
  line L2 (-13, 23) -> (13, 23)
  line L3 (13, 23) -> (13, -23)
  circle A0 centre (-10, 10) radius 1.5
  circle A1 centre (10, 10) radius 1.5
  circle A2 centre (-10, -10) radius 1.5
  circle A3 centre (10, -10) radius 1.5
  point P0 (-10, 10)
  point P1 (10, 10)
  point P2 (10, -10)
  point P3 (-10, -10)
  dimension "d1" = 26
  dimension "d2" = 46
  dimension "d3" = 20
  dimension "d4" = 20
  dimension "d5" = 3
  dimension "d6" = 3
  dimension "d7" = 3
  dimension "d8" = 3
  constraint perpendicular L0 L1
  constraint parallel L0 L2
  constraint parallel L1 L3
  constraint horizontal L0
  constraint coincident P0 A0.centre
  constraint coincident P1 A1.centre
  constraint coincident P3 A2.centre
  constraint coincident P2 A3.centre
  measures "d1" distance of L1.end L2.end
  measures "d2" distance of L0.end L1.end
  measures "d3" distance of P0 P1
  measures "d4" distance of P0 P3
  measures "d5" diameter of A0
  measures "d6" diameter of A1
  measures "d7" diameter of A2
  measures "d8" diameter of A3
extrude "Extrude1" add sketch "Sketch1" along normal blind 9.525

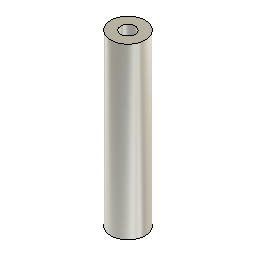
design "long stepper tube"
Autodesk Fusion 360 part; units mm, degrees
sketch "Sketch1" plane through (0, 0, 0) normal (0, 0, 1) x (1, 0, 0)
  circle A0 centre (0, 0) radius 6
  circle A1 centre (0, 0) radius 2.5
  dimension "d1" = 12
  dimension "d2" = 5
  constraint coincident A0.centre A1.centre
  measures "d1" diameter of A0
  measures "d2" diameter of A1
extrude "Extrude1" add sketch "Sketch1" along normal blind 59
ref_plane "WorkPlane1" through (0, 0, 0) normal (0, 1, 0) x (0, 0, 1)
sketch "Sketch2" plane through (0, 0, 0) normal (0, 1, 0) x (1, 0, 0)
  line L0 (-6, -59) -> (-6, 0)
  constraint vertical L0
ref_plane "WorkPlane2" through (0, 0, 0) normal (0, 1, 0) x (0, 0, 1)
sketch "Sketch3" plane through (0, 0, 0) normal (0, 1, 0) x (1, 0, 0)
  line L0 (-6, 0) -> (-6, -59)
  point P0 (-6, 0)
  point P1 (-6, -59)
  constraint coincident P0 L0.start
  constraint coincident P1 L0.end

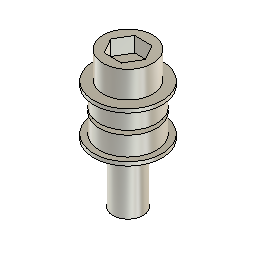
design "8mm bridge pulley"
Autodesk Fusion 360 part; units mm, degrees
sketch "Sketch1" plane through (0, 0, 0) normal (0, 0, 1) x (1, 0, 0)
sketch "Sketch2" plane through (0, 0, 0) normal (0, 0, 1) x (1, 0, 0)
  circle A0 centre (0, 0) radius 4
  dimension "d4" = 8
  constraint coincident A0.centre origin
  measures "d4" diameter of A0
extrude "Extrude2" add sketch "Sketch2" along normal blind 27 makes body 1
sketch "Sketch3" plane through (0, 0, 27) normal (0, 0, 1) x (-1, 0, 0)
  circle A0 centre (0, 0) radius 4
  circle A1 centre (0, 0) radius 6.5
  dimension "d7" = 13
  constraint concentric A0 A1
  measures "d7" diameter of A1
extrude "Extrude3" add sketch "Sketch3" along normal blind 10 contours A0 | A1 bodies 1
sketch "Sketch4" plane through (0, 0, 37) normal (0, 0, 1) x (-1, 0, 0)
  circle A0 centre (0, 0) radius 6.5
  line L0 (-4.6182, 0.0754) -> (-2.3744, -3.9618)
  line L1 (-2.3744, -3.9618) -> (2.2438, -4.0372)
  line L2 (2.2438, -4.0372) -> (4.6182, -0.0754)
  line L3 (4.6182, -0.0754) -> (2.3744, 3.9618)
  line L4 (2.3744, 3.9618) -> (-2.2438, 4.0372)
  line L5 (-2.2438, 4.0372) -> (-4.6182, 0.0754)
  dimension "d10" = 4
  constraint coincident A0.centre origin
  measures "d10" distance of A0.centre L5
extrude "Extrude4" cut sketch "Sketch4" against normal blind 7 contours L0 L1 L2 L3 L4 L5 bodies 1
thread "Thread1" [suppressed]
sketch "Sketch5" plane through (0, 0, 37) normal (0, 0, 1) x (-1, 0, 0)
  circle A0 centre (-1.5099, 25.9558) radius 4
  circle A1 centre (-1.5099, 25.9558) radius 8
  circle A2 centre (-1.5099, 25.9558) radius 9
  dimension "d13" = 8
  dimension "d14" = 16
  dimension "d15" = 18
  constraint concentric A0 A1
  constraint concentric A1 A2
  measures "d13" diameter of A0
  measures "d14" diameter of A1
  measures "d15" diameter of A2
sketch "Sketch6" plane through (0, 0, 42) normal (0, 0, 1) x (-1, 0, 0)
  circle A0 centre (-1.5099, 25.9558) radius 4
  circle A1 centre (-1.5099, 25.9558) radius 8
  circle A2 centre (-1.5099, 25.9558) radius 5
  circle A3 centre (-1.5099, 25.9558) radius 7.5
  dimension "d20" = 10
  dimension "d21" = 15
  constraint concentric A0 A2
  constraint concentric A2 A3
  measures "d20" diameter of A2
  measures "d21" diameter of A3
extrude "Extrude7" add sketch "Sketch6" against normal blind 5 separate body contours A3 makes body 2
extrude "Extrude8" add sketch "Sketch5" against normal blind 1 separate body contours A2 makes body 3
sketch "Sketch7" plane through (0, 0, 42) normal (0, 0, 1) x (1, 0, 0)
extrude "Extrude9" add sketch "Sketch5" against normal blind 1 contours A1 bodies 2 3
move_face "OffsetFaces1" offset 5 1 faces at (-3.1382, -25.7074, 37) on bodies 2
copy_body "CopyPasteBodies1" bodies 2 makes body 4
move_body "Move1" bodies 4 to x (-1, 0, 0) y (0, 1, 0) z (0, 0, -1) at (3.0197, 0, 84.5)
move_body "Move2" bodies 1 to x (1, 0, 0) y (0, 1, 0) z (0, 0, 1) at (44, -25, 0)
move_body "Align1" bodies 1 to x (1, 0, 0) y (0, 1, 0) z (0, 0, 1) at (-42.4901, -0.9558, 45.7324)
move_body "Move3" bodies 2 4 to x (1, 0, 0) y (0, 1, 0) z (0, 0, 1) at (0, 0, 24)
move_body "Move4" bodies 2 to x (1, 0, 0) y (0, 1, 0) z (0, 0, 1) at (0, 0, -55)
sketch "Sketch8" plane through (0, 0, 45.7324) normal (0, 0, -1) x (1, 0, 0)
  circle A0 centre (1.5091, 25.9519) radius 4
  circle A1 centre (1.5091, 25.9519) radius 5
  circle A2 centre (1.5099, 25.9558) radius 4
  dimension "d29" = 8
  dimension "d30" = 10
  constraint concentric A0 A1
  measures "d29" diameter of A0
  measures "d30" diameter of A1
extrude "Extrude10" add sketch "Sketch6" along normal blind 1 separate body contours A2 makes body 5
move_body "Move5" bodies 5 to x (1, 0, 0) y (0, 1, 0) z (0, 0, 1) at (0, 0, 23.5)
move_body "Move6" bodies 2 to x (1, 0, 0) y (0, 1, 0) z (0, 0, 1) at (0, 0, 54.4)
sketch "Sketch9" plane through (0, 0, 45.7324) normal (0, 0, -1) x (1, 0, 0)
  circle A0 centre (1.5097, 25.9553) radius 4
  circle A1 centre (1.5097, 25.9553) radius 5
  circle A2 centre (1.5099, 25.9558) radius 4
  dimension "d34" = 8
  dimension "d35" = 10
  constraint concentric A0 A1
  measures "d34" diameter of A0
  measures "d35" diameter of A1
extrude "Extrude11" add sketch "Sketch8" against normal blind 10 separate body makes body 6
move_body "Move7" bodies 6 to x (1, 0, 0) y (0, 1, 0) z (0, 0, 1) at (0, 0, 3.5)
move_face "OffsetFaces3" offset -9 1 faces at (-0.5142, -21.7571, 49.2324) on bodies 6
extrude "Extrude12" cut 1 faces at (1.7153, -21.1289, 82.7324) along direction (0, 0, -1) blind 3 on bodies 1 bodies 1
move_face "OffsetFaces4" offset 2 1 faces at (2.8836, -26.8924, 45.7324) on bodies 1
move_face "OffsetFaces5" offset 0.7 1 faces at (6.4843, -25.4541, 58.8991) on bodies 6
combine "Combine1" [suppressed]
named bodies: "pulley low"

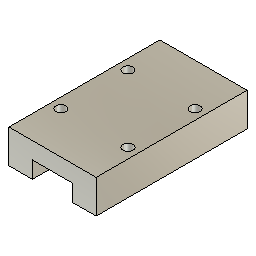
design "rail block"
Autodesk Fusion 360 part; units mm, degrees
sketch "Sketch1" plane through (0, 0, 0) normal (0, 1, 0) x (1, 0, 0)
  line L0 (-13, 5) -> (-13, -5)
  line L1 (-13, -5) -> (13, -5)
  line L2 (13, -5) -> (13, 5)
  line L3 (13, 5) -> (-13, -5) construction
  line L4 (-13, 5) -> (13, -5) construction
  line L5 (0, 0) -> (6, 0)
  line L6 (6, 0) -> (6, 5)
  line L7 (0, 0) -> (-6, 0)
  line L8 (-6, 0) -> (-6, 5)
  line L9 (13, 5) -> (6, 5)
  line L10 (-6, 5) -> (-13, 5)
  dimension "d1" = 26
  dimension "d2" = 10
  dimension "d5" = 6
  dimension "d6" = 6
  constraint perpendicular L0 L9
  constraint parallel L1 L9
  constraint parallel L0 L2
  constraint horizontal L9
  constraint coincident L3 L5.start
  constraint coincident L4 L5.start
  constraint coincident L5.start L7.start
  constraint perpendicular L0 L5
  constraint perpendicular L6 L9
  constraint perpendicular L6 L7
  constraint coincident L8.end L9
  constraint perpendicular L8 L9
  constraint collinear L9 L10
  measures "d1" distance of L0.end L1.end L2.end
  measures "d2" distance of L0.start L0.end
  measures "d5" distance of L5.start L5.end
  measures "d6" distance of L5.start L7.end
extrude "Extrude1" add sketch "Sketch1" along normal blind 45
sketch "Sketch2" plane through (0, 0, 5) normal (0, 0, 1) x (-1, 0, 0)
  line L0 (13, 0) -> (-13, 0)
  line L1 (-13, 0) -> (-13, -45)
  line L2 (-13, -45) -> (13, -45)
  line L3 (13, -45) -> (13, 0)
  circle A0 centre (10, -32.5) radius 1.5
  circle A1 centre (10, -12.5) radius 1.5
  circle A2 centre (-10, -32.5) radius 1.5
  circle A3 centre (-10, -12.5) radius 1.5
  point P0 (0, -22.5)
  point P1 (10, -32.5)
  point P2 (-10, -32.5)
  point P3 (-10, -12.5)
  point P4 (10, -12.5)
  dimension "d7" = 20
  dimension "d8" = 20
  dimension "d9" = 3
  dimension "d10" = 3
  dimension "d11" = 3
  dimension "d12" = 3
  constraint coincident P1 A0.centre
  constraint coincident P2 A2.centre
  constraint coincident P3 A3.centre
  constraint coincident P4 A1.centre
  measures "d7" distance of P1 P4
  measures "d8" distance of P1 P2
  measures "d9" diameter of A0
  measures "d10" diameter of A1
  measures "d11" diameter of A2
  measures "d12" diameter of A3
hole "Hole1" at (-10, 32.5, 5) direction (0, 0, -1) diameter 3 depth 8 tip angle 118
hole "Hole2" at (10, 32.5, 5) at (10, 12.5, 5) at (-10, 12.5, 5) direction (0, 0, -1) diameter 3 depth 8 tip angle 118

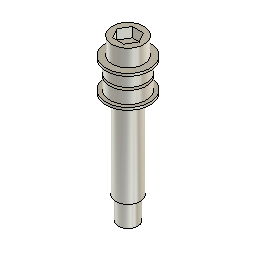
design "8mm pulley high"
Autodesk Fusion 360 part; units mm, degrees
sketch "Sketch1" plane through (0, 0, 0) normal (0, 0, 1) x (1, 0, 0)
sketch "Sketch2" plane through (0, 0, 0) normal (0, 0, 1) x (1, 0, 0)
  circle A0 centre (0, 0) radius 4
  dimension "d4" = 8
  constraint coincident A0.centre origin
  measures "d4" diameter of A0
extrude "Extrude2" add sketch "Sketch2" along normal blind 27 contours A0 picked at (1.42018, -0.528552) makes body 1
sketch "Sketch3" plane through (0, 0, 27) normal (0, 0, 1) x (-1, 0, 0)
  circle A0 centre (0, 0) radius 4
  circle A1 centre (0, 0) radius 6.5
  dimension "d7" = 13
  constraint concentric A0 A1
  measures "d7" diameter of A1
extrude "Extrude3" add sketch "Sketch3" along normal blind 10 contours A0 | A1 picked at (-0.705317, 0.780795) picked at (5.627575, -0.521648) bodies 1
sketch "Sketch4" plane through (0, 0, 37) normal (0, 0, 1) x (-1, 0, 0)
  circle A0 centre (0, 0) radius 6.5
  line L0 (-4.618187, 0.0754) -> (-2.374392, -3.961767)
  line L1 (-2.374392, -3.961767) -> (2.243795, -4.037167)
  line L2 (2.243795, -4.037167) -> (4.618187, -0.0754)
  line L3 (4.618187, -0.0754) -> (2.374392, 3.961767)
  line L4 (2.374392, 3.961767) -> (-2.243795, 4.037167)
  line L5 (-2.243795, 4.037167) -> (-4.618187, 0.0754)
  dimension "d10" = 4
  constraint coincident A0.centre origin
  measures "d10" distance of A0.centre L5
extrude "Extrude4" cut sketch "Sketch4" against normal blind 7 contours L0 L1 L2 L3 L4 L5 picked at (-1.539396, 0.025133) bodies 1
thread "Thread1" [suppressed]
sketch "Sketch5" plane through (0, 0, 37) normal (0, 0, 1) x (-1, 0, 0)
  circle A0 centre (-1.50985, 25.955849) radius 4
  circle A1 centre (-1.50985, 25.955849) radius 8
  circle A2 centre (-1.50985, 25.955849) radius 9
  dimension "d13" = 8
  dimension "d14" = 16
  dimension "d15" = 18
  constraint concentric A0 A1
  constraint concentric A1 A2
  measures "d13" diameter of A0
  measures "d14" diameter of A1
  measures "d15" diameter of A2
sketch "Sketch6" plane through (0, 0, 42) normal (0, 0, 1) x (-1, 0, 0)
  circle A0 centre (-1.50985, 25.955849) radius 4
  circle A1 centre (-1.50985, 25.955849) radius 8
  circle A2 centre (-1.50985, 25.955849) radius 5
  circle A3 centre (-1.50985, 25.955849) radius 7.5
  dimension "d20" = 10
  dimension "d21" = 15
  constraint concentric A0 A2
  constraint concentric A2 A3
  measures "d20" diameter of A2
  measures "d21" diameter of A3
extrude "Extrude7" add sketch "Sketch6" against normal blind 5 separate body contours A3 picked at (5.110278, 25.33484) makes body 2
extrude "Extrude8" add sketch "Sketch5" against normal blind 1 separate body contours A2 picked at (7.093525, 25.111277) makes body 3
sketch "Sketch7" plane through (0, 0, 42) normal (0, 0, 1) x (1, 0, 0)
extrude "Extrude9" add sketch "Sketch5" against normal blind 1 contours A1 picked at (5.11214, 25.35968) bodies 2 3
move_face "OffsetFaces1" offset 5 1 faces at (-3.138201, -25.707446, 37) on bodies 2
copy_body "CopyPasteBodies1" bodies 2 makes body 4
move_body "Move1" bodies 4 to x (-1, 0, 0) y (0, 1, 0) z (0, 0, -1) at (3.0197, 0, 84.5)
move_body "Move2" bodies 1 to x (1, 0, 0) y (0, 1, 0) z (0, 0, 1) at (44, -25, 0)
move_body "Align1" bodies 1 to x (1, 0, 0) y (0, 1, 0) z (0, 0, 1) at (-42.49015, -0.955849, 45.732394)
move_body "Move3" bodies 2 4 to x (1, 0, 0) y (0, 1, 0) z (0, 0, 1) at (0, 0, 24)
move_body "Move4" bodies 2 to x (1, 0, 0) y (0, 1, 0) z (0, 0, 1) at (0, 0, -55)
sketch "Sketch8" plane through (0, 0, 45.732394) normal (0, 0, -1) x (1, 0, 0)
  circle A0 centre (1.50914, 25.951936) radius 4
  circle A1 centre (1.50914, 25.951936) radius 5
  circle A2 centre (1.50985, 25.955849) radius 4
  dimension "d29" = 8
  dimension "d30" = 10
  constraint concentric A0 A1
  measures "d29" diameter of A0
  measures "d30" diameter of A1
extrude "Extrude10" add sketch "Sketch6" along normal blind 1 separate body contours A2 picked at (3.138201, 25.707446) makes body 5
move_body "Move5" bodies 5 to x (1, 0, 0) y (0, 1, 0) z (0, 0, 1) at (0, 0, 23.5)
move_body "Move6" bodies 2 to x (1, 0, 0) y (0, 1, 0) z (0, 0, 1) at (0, 0, 54.4)
sketch "Sketch9" plane through (0, 0, 45.732394) normal (0, 0, -1) x (1, 0, 0)
  circle A0 centre (1.50974, 25.955286) radius 4
  circle A1 centre (1.50974, 25.955286) radius 5
  circle A2 centre (1.50985, 25.955849) radius 4
  dimension "d34" = 8
  dimension "d35" = 10
  constraint concentric A0 A1
  measures "d34" diameter of A0
  measures "d35" diameter of A1
extrude "Extrude11" add sketch "Sketch8" against normal blind 10 separate body contours A1 picked at (-0.514215, 21.757072) makes body 6
move_body "Move7" bodies 6 to x (1, 0, 0) y (0, 1, 0) z (0, 0, 1) at (0, 0, 3.5)
move_face "OffsetFaces3" offset -3 1 faces at (-0.514215, -21.757072, 49.232394) on bodies 6
extrude "Extrude12" cut 1 faces at (1.715297, -21.12893, 82.732394) along direction (0, 0, -1) blind 3 on bodies 1 bodies 1
move_face "OffsetFaces4" offset 21 1 faces at (2.883587, -26.892448, 45.732394) on bodies 1
extrude "Extrude13" add 1 faces at (-0.514215, -21.757072, 52.232394) along direction (0, 0, -1) blind 17 on bodies 6 bodies 6 2 4 5 1